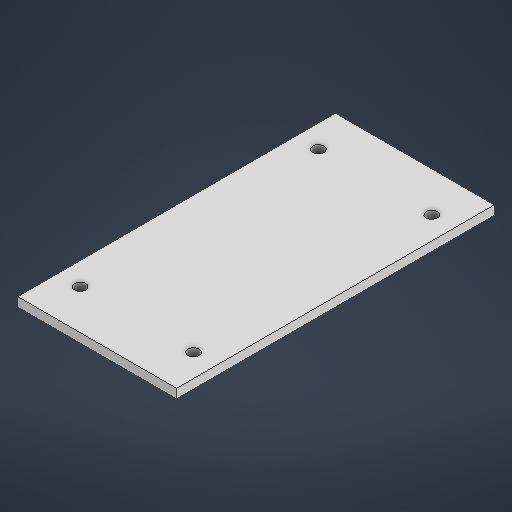
# Autodesk Inventor part: rackmountplate
Saved by Autodesk Inventor 2026.2 (Build 302298010, 298A)
## iProperties
Created: 2026-07-06
Part Number: rackmountplate
Material: Generic
Document SubType Name: Modeling
Designer: tasle
Density: 1 g/cm^3
Appearance: Default
Author: tasle
Autodesk Inventor part; units mm, degrees
ref_plane "YZ Plane" through (0, 0, 0) normal (1, 0, 0) x (0, 1, 0)
ref_plane "XZ Plane" through (0, 0, 0) normal (0, 1, 0) x (-1, 0, 0)
ref_plane "XY Plane" through (0, 0, 0) normal (0, 0, 1) x (1, 0, 0)
sketch "Sketch1" plane through (0, 0, 0) normal (0, 1, 0) x (-1, 0, 0)
  line L0 (1.6562, 11.8846) -> (-68.3438, 11.8846)
  line L1 (-68.3438, 11.8846) -> (-68.3438, -128.1154)
  line L2 (-68.3438, -128.1154) -> (1.6562, -128.1154)
  line L3 (1.6562, -128.1154) -> (1.6562, 11.8846)
  line L4 (-8.3438, -5.6154) -> (-58.3438, -5.6154)
  line L5 (-58.3438, -5.6154) -> (-58.3438, -110.6154)
  line L6 (-58.3438, -110.6154) -> (-8.3438, -110.6154)
  line L7 (-8.3438, -110.6154) -> (-8.3438, -5.6154)
  circle A0 centre (-8.3438, -5.6154) radius 2.5
  circle A1 centre (-8.3438, -110.6154) radius 2.5
  circle A2 centre (-58.3438, -5.6154) radius 2.5
  circle A3 centre (-58.3438, -110.6154) radius 2.5
  point P0 (0, 0)
  dimension "d0" = 70
  dimension "d1" = 140
  dimension "d2" = 50
  dimension "d3" = 105
  dimension "d4" = 17.5
  dimension "d5" = 10
  dimension "d6" = 5
  dimension "d7" = 5
  dimension "d8" = 5
  dimension "d9" = 5
  constraints: 16 end point, 4 centre point, 4 coincident, 4 parallel, 2 horizontal, 2 perpendicular
  measures "d0" distance of L2.end L1.end
  measures "d1" distance of L1.end L0.end
  measures "d2" distance of L6.end L5.end
  measures "d3" distance of L5.end L4.end
  measures "d4" distance between parallel lines of L2 L6
  measures "d5" distance between parallel lines of L3 L7
  measures "d6" diameter of A0
  measures "d7" diameter of A1
  measures "d8" diameter of A2
  measures "d9" diameter of A3
extrude "Extrusion1" add sketch "Sketch1" along normal blind 4 contours L3 L2 L1 L0 | L4 A0 L7 A1 L6 A3 L5 A2
body "Solid1"
